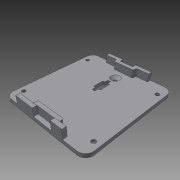
# Autodesk Inventor part: top
Saved by Autodesk Inventor 2014 (Build 180170000, 170)
## iProperties
Created: 2015-11-09
Part Number: top
Material: Generic
Document SubType Name: Modeling
Designer: buben
Density: 1 g/cm^3
Appearance: Default
Author: buben
Autodesk Inventor part; units mm, degrees
ref_plane "YZ Plane" through (0, 0, 0) normal (1, 0, 0) x (0, 1, 0)
ref_plane "XZ Plane" through (0, 0, 0) normal (0, 1, 0) x (-1, 0, 0)
ref_plane "XY Plane" through (0, 0, 0) normal (0, 0, 1) x (1, 0, 0)
sketch "Sketch1" plane through (0, 0, 0) normal (0, 1, 0) x (-1, 0, 0)
  line L0 (0, 0) -> (-70, 0)
  line L1 (-70, 0) -> (-70, -76)
  line L2 (-70, -76) -> (0, -76)
  line L3 (0, -76) -> (0, 0)
  dimension "d0" = 70
  dimension "d1" = 76
  constraints: 8 end point, 2 parallel, 1 horizontal, 1 perpendicular
  measures "d0" distance of L0.start L0.end
  measures "d1" distance between parallel lines of L0 L2
extrude "Extrusion1" add sketch "Sketch1" along normal blind 3
sketch "Sketch2" plane through (0, 3, 0) normal (0, 1, 0) x (1, 0, 0)
  line L0 (70, 76) -> (0, 76) projected
  line L1 (16.33, 76) -> (30.05, 76)
  line L2 (30.05, 76) -> (30.05, 73)
  line L3 (30.05, 73) -> (16.33, 73)
  line L4 (16.33, 73) -> (16.33, 76)
  line L5 (39.95, 76) -> (53.67, 76)
  line L6 (53.67, 76) -> (53.67, 73)
  line L7 (53.67, 73) -> (39.95, 73)
  line L8 (39.95, 73) -> (39.95, 76)
  line L9 (30.05, 74.5) -> (39.95, 74.5) construction
  line L10 (0, 76) -> (0, 0) projected
  point P0 (23.19, 73)
  point P1 (46.81, 73)
  point P2 (35, 74.5)
  point P3 (35, 76)
  dimension "d4" = 13.72
  dimension "d5" = 13.72
  dimension "d6" = 3
  dimension "d29" = 16.33
  constraints: 18 end point, 6 midpoint, 4 parallel, 2 horizontal, 2 perpendicular, 2 point on line, 1 collinear, 1 vertical alignment
  measures "d4" distance of L2.end L3.end
  measures "d5" distance of L6.end L7.end
  measures "d6" distance of L3.end L1.start
  measures "d29" distance between parallel lines of L10 L4
extrude "Extrusion2" add sketch "Sketch2" along normal blind 6.3
sketch "Sketch3" plane through (0, 3, 0) normal (0, 1, 0) x (1, 0, 0)
  line L0 (0, 0) -> (70, 0) projected
  line L1 (44.67, 0) -> (53.67, 0)
  line L2 (53.67, 0) -> (53.67, 3)
  line L3 (53.67, 3) -> (44.67, 3)
  line L4 (44.67, 3) -> (44.67, 0)
  line L5 (53.67, 76) -> (53.67, 73) projected
  dimension "d10" = 9
  dimension "d11" = 3
  constraints: 8 end point, 2 parallel, 1 collinear, 1 horizontal, 1 perpendicular, 1 point on line
  measures "d10" distance of L2.end L3.end
  measures "d11" distance of L3.end L1.start
extrude "Extrusion3" add sketch "Sketch3" along normal blind 7.1
sketch "Sketch4" plane through (0, 3, 0) normal (0, 1, 0) x (1, 0, 0)
  line L0 (16.33, 73) -> (16.33, 76) projected
  line L1 (0, 0) -> (44.67, 0) projected
  line L2 (44.67, 0) -> (44.67, 3) projected
  line L3 (12.87, 0) -> (28.97, 0)
  line L4 (28.97, 0) -> (28.97, 3)
  line L5 (28.97, 3) -> (12.87, 3)
  line L6 (12.87, 3) -> (12.87, 0)
  dimension "d16" = 16.1
  dimension "d17" = 15.7
  constraints: 8 end point, 3 parallel, 1 horizontal, 1 perpendicular, 1 point on line
  measures "d16" distance of L4.end L5.end
  measures "d17" distance between parallel lines of L2 L4
extrude "Extrusion4" add sketch "Sketch4" along normal blind 6.2
sketch "Sketch5" plane through (0, 0, 0) normal (0, -1, 0) x (1, 0, 0)
  line L0 (0, 0) -> (70, 0) projected
  line L1 (0, -76) -> (0, 0) projected
  line L2 (4.5, -10) -> (65.5, -10) construction
  line L3 (65.5, -10) -> (65.5, -66) construction
  line L4 (65.5, -66) -> (4.5, -66) construction
  line L5 (4.5, -66) -> (4.5, -10) construction
  point P0 (35, -10)
  point P1 (35, 0)
  point P2 (4.5, -38)
  point P3 (0, -38)
  dimension "d20" = 10
  dimension "d21" = 4.5
  constraints: 8 end point, 4 coincident, 4 midpoint, 2 parallel, 1 horizontal, 1 horizontal alignment, 1 perpendicular, 1 vertical alignment
  measures "d20" distance between parallel lines of L0 L2
  measures "d21" distance between parallel lines of L1 L5
hole "Hole1" at (4.5, 0, -10) at (4.5, 0, -66) at (65.5, 0, -66) at (65.5, 0, -10) direction (0, 1, 0) diameter 3.2 end through all counterbore diameter 6 counterbore depth 1
fillet "Fillet1" radius 6 4 edges at (0, 1.5, 0) (70, 1.5, 0) (70, 1.5, -76) (0, 1.5, -76)
sketch "Sketch6" plane through (0, 3, 0) normal (0, 1, 0) x (1, 0, 0)
  line L0 (16.33, 76) -> (6, 76) projected
  line L1 (13.03, 69.24) -> (56.97, 69.24) construction
  line L2 (0, 70) -> (70, 70) construction
  line L3 (13.03, 69.24) -> (13.03, 6.76) construction
  line L4 (6, 76) -> (6, 0) construction
  line L5 (37.62, 53.42) -> (37.62, 44.42)
  line L6 (31.62, 44.42) -> (31.62, 53.42)
  line L7 (33.37, 56.42) -> (35.87, 56.42)
  line L8 (35.87, 41.42) -> (33.37, 41.42)
  line L9 (31.62, 53.42) -> (33.37, 53.42)
  line L10 (35.87, 53.42) -> (37.62, 53.42)
  line L11 (37.62, 44.42) -> (35.87, 44.42)
  line L12 (33.37, 44.42) -> (31.62, 44.42)
  line L13 (33.37, 41.42) -> (33.37, 44.42)
  line L14 (33.37, 53.42) -> (33.37, 56.42)
  line L15 (35.87, 56.42) -> (35.87, 53.42)
  line L16 (35.87, 44.42) -> (35.87, 41.42)
  circle A0 centre (35.13, 61.87) radius 1.5
  point P0 (0, 0)
  point P1 (35, 69.24)
  point P2 (35, 70)
  point P3 (6, 38)
  point P4 (13.03, 38)
  point P5 (34.62, 56.42)
  point P6 (31.62, 48.92)
  dimension "d31" = 43.94
  dimension "d32" = 62.48
  dimension "d33" = 6
  dimension "d34" = 9
  dimension "d35" = 2.5
  dimension "d36" = 15
  dimension "d38" = 20.32
  dimension "d39" = 3
  dimension "d40" = 7.37
  dimension "d44" = 21.84
  dimension "d45" = 22.35
  constraints: 32 end point, 13 parallel, 6 collinear, 6 midpoint, 5 perpendicular, 3 horizontal, 1 centre point, 1 horizontal alignment, 1 vertical alignment
  measures "d31" distance of L1.start L1.end
  measures "d32" distance of L1.start L3.end
  measures "d33" distance between parallel lines of L5 L6
  measures "d34" distance of L6.start L6.end
  measures "d35" distance of L7.start L7.end
  measures "d36" distance between parallel lines of L8 L7
  measures "d38" vertical distance of L1.start point (31.62, 48.92)
  measures "d39" diameter of A0
  measures "d40" vertical distance of A0.centre L1.start
  measures "d44" horizontal distance of L1.end A0.centre
  measures "d45" horizontal distance of L1.end point (34.62, 56.42)
extrude "Extrusion5" cut sketch "Sketch6" against normal through all
fillet "Fillet2" radius 0.5 12 edges at (35.87, 1.5, -53.42) (33.37, 1.5, -53.42) (35.87, 1.5, -56.42) (33.37, 1.5, -56.42) (37.62, 1.5, -53.42) (37.62, 1.5, -44.42) (35.87, 1.5, -44.42) (35.87, 1.5, -41.42) (33.37, 1.5, -41.42) (33.37, 1.5, -44.42) (31.62, 1.5, -44.42) (31.62, 1.5, -53.42)
chamfer "Chamfer1" distance 2.5 angle 45 1 edges at (33.63, 3, -61.87)
sketch "Sketch7" plane through (30.05, 9.3, -76) normal (0, 0, -1) x (-1, 0, 0)
  line L0 (-9.9, -6.3) -> (-9.9, 0) projected
  line L1 (-23.62, 0) -> (-9.9, 0) projected
  line L2 (-33.95, -6.3) -> (-23.62, -6.3) projected
  line L3 (-23.62, 0) -> (-23.12, 0)
  line L4 (-23.12, 0) -> (-23.12, -6.3)
  line L5 (-23.12, -6.3) -> (-23.62, -6.3)
  line L6 (-23.62, -6.3) -> (-23.62, 0)
  line L7 (-10.4, 0) -> (-9.9, 0)
  line L8 (-9.9, 0) -> (-9.9, -6.3)
  line L9 (-9.9, -6.3) -> (-10.4, -6.3)
  line L10 (-10.4, -6.3) -> (-10.4, 0)
  line L11 (0, 0) -> (0.5, 0)
  line L12 (0.5, 0) -> (0.5, -6.3)
  line L13 (0.5, -6.3) -> (0, -6.3)
  line L14 (0, -6.3) -> (0, 0)
  line L15 (13.72, 0) -> (13.22, 0)
  line L16 (13.22, 0) -> (13.22, -6.3)
  line L17 (13.22, -6.3) -> (13.72, -6.3)
  line L18 (13.72, -6.3) -> (13.72, 0)
  point P0 (30.05, -9.3)
  dimension "d50" = 0.5
  constraints: 32 end point, 8 parallel, 6 collinear, 4 horizontal, 4 perpendicular, 1 point on line
  measures "d50" distance of L4.end L5.end
extrude "Extrusion6" cut sketch "Sketch7" against normal up to surface (3 mm away)
sketch "Sketch8" plane through (0, 3, 0) normal (0, 1, 0) x (1, 0, 0)
  line L0 (12.87, 3) -> (28.97, 3) projected
  line L1 (44.67, 0) -> (44.67, 3) projected
  line L2 (44.67, 3) -> (53.67, 3) projected
  line L3 (53.17, 73) -> (40.45, 73) projected
  line L4 (29.55, 73) -> (16.83, 73) projected
  line L5 (33.37, 41.92) -> (33.37, 43.92) projected
  line L6 (28.97, 3) -> (28.97, 3.2)
  line L7 (28.97, 3.2) -> (44.67, 3.2)
  line L8 (44.67, 3.2) -> (44.67, 3)
  line L9 (28.97, 3) -> (25.97, 3)
  line L10 (25.97, 3) -> (25.97, 6.2)
  line L11 (25.97, 6.2) -> (47.67, 6.2)
  line L12 (47.67, 6.2) -> (47.67, 3)
  line L13 (47.67, 3) -> (44.67, 3)
  line L14 (29.55, 73) -> (29.55, 72.8)
  line L15 (29.55, 72.8) -> (40.45, 72.8)
  line L16 (40.45, 72.8) -> (40.45, 73)
  line L17 (40.45, 73) -> (43.45, 73)
  line L18 (43.45, 73) -> (43.45, 69.8)
  line L19 (43.45, 69.8) -> (26.55, 69.8)
  line L20 (26.55, 69.8) -> (26.55, 73)
  line L21 (26.55, 73) -> (29.55, 73)
  point P0 (0, 0)
  dimension "d53" = 0.2
  dimension "d54" = 3
  dimension "d55" = 3
  dimension "d56" = 3
  dimension "d57" = 3
  dimension "d58" = 3
  dimension "d59" = 3
  constraints: 32 end point, 9 perpendicular, 5 parallel, 4 point on line, 1 collinear
  measures "d53" distance of L4.start L14.end
  measures "d54" distance between parallel lines of L15 L19
  measures "d55" horizontal distance of L14.end L19.end
  measures "d56" horizontal distance of L18.end L15.end
  measures "d57" distance between parallel lines of L11 L7
  measures "d58" horizontal distance of L10.end L6.end
  measures "d59" horizontal distance of L7.end L11.end
extrude "Extrusion7" add sketch "Sketch8" along normal up to surface (6.3 mm away)
fillet "Fillet3" radius 0.5 4 edges at (29.55, 6.15, -72.8) (40.45, 6.15, -72.8) (44.67, 6.15, -3.2) (28.97, 6.15, -3.2)
fillet "Fillet4" radius 1 8 edges at (43.45, 6.15, -73) (43.45, 6.15, -69.8) (26.55, 6.15, -73) (26.55, 6.15, -69.8) (47.67, 6.15, -3) (47.67, 6.15, -6.2) (25.97, 6.1, -3) (25.97, 6.15, -6.2)
equation "\"d5\" = d4"
equation "\"d55\" = d54"
equation "\"d56\" = d55"
equation "\"d57\" = d54"
equation "\"d58\" = d57"
equation "\"d59\" = d57"
body "Solid1"
